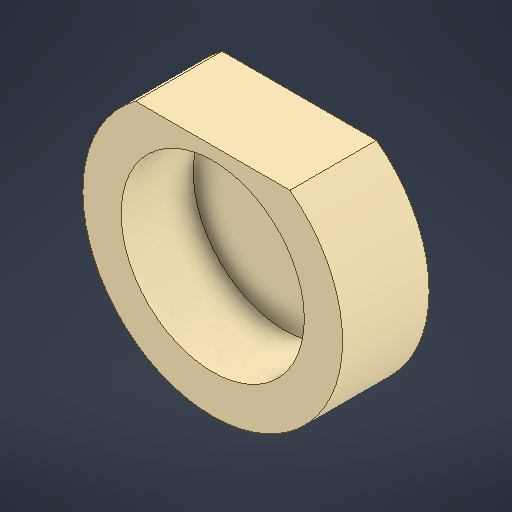
# Autodesk Inventor part: Miska
Saved by Autodesk Inventor 2026.1 (Build 301233000, 233)
## iProperties
Created: 2025-09-11
Part Number: Miska
Material: Všeobecné
Document SubType Name: Modeling
Designer: cerna
Density: 1 g/cm^3
Appearance: Béžová
Author: cerna
Autodesk Inventor part; units mm, degrees
ref_plane "YZ Plane" through (0, 0, 0) normal (1, 0, 0) x (0, 1, 0)
ref_plane "XZ Plane" through (0, 0, 0) normal (0, 1, 0) x (-1, 0, 0)
ref_plane "XY Plane" through (0, 0, 0) normal (0, 0, 1) x (1, 0, 0)
sketch "Náčrt1" plane through (0, 0, 0) normal (0, 0, 1) x (1, 0, 0)
  line L0 (0, 104.8468) -> (0, -122.4745) projected
  line L1 (-126, 0) -> (126, 0) projected
  circle A0 centre (0, 0) radius 63.5
  arc A1 (-53.5, 72.3723) -> (53.5, 72.3723) centre (0, 0) ccw
  line L2 (-53.5, 72.3723) -> (53.5, 72.3723)
  dimension "d0" = 127
  dimension "d1" = 180
  dimension "d2" = 107
  constraints: 2 centre point, 2 coincident, 2 end point, 2 point on circle, 1 horizontal
  measures "d0" diameter of A0
  measures "d1" diameter of A1
  measures "d2" distance of L2.start L2.end
extrude "Vysunutí1" add sketch "Náčrt1" along normal blind 10
sketch "Náčrt2" plane through (0, 0, 10) normal (0, 0, 1) x (1, 0, 0)
  circle A0 centre (0, 0) radius 63.5
  line L0 (53.5, 72.3723) -> (-53.5, 72.3723) projected
  arc A1 (-53.5, 72.3723) -> (53.5, 72.3723) centre (0, 0) ccw projected
  arc A2 (-53.5, 72.3723) -> (53.5, 72.3723) centre (0, 0) ccw
  line L1 (-53.5, 72.3723) -> (53.5, 72.3723)
  dimension "d5" = 127
  constraints: 2 centre point, 2 coincident, 2 end point, 2 point on circle, 1 collinear, 1 concentric
  measures "d5" diameter of A0
extrude "Vysunutí2" add sketch "Náčrt2" along normal blind 50
